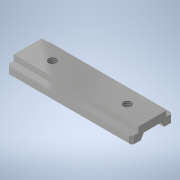
# Autodesk Inventor part: MR-20CS
Saved by Autodesk Inventor 2022 (Build 260153000, 153)
## iProperties
Created: 2022-02-08
Part Number: MR-20CS
Material: ポリエチレン、高密度
Document SubType Name: Modeling
Designer: satot
Density: 0.952 g/cm^3
Appearance: 滑らか - 標準の灰色
Mass: 2.70649 g
Surface Area: 24.218 cm^2
Volume: 2.84295 cm^3
Author: satot
Autodesk Inventor part; units mm, degrees
ref_plane "YZ Plane" through (0, 0, 0) normal (1, 0, 0) x (0, 1, 0)
ref_plane "XZ Plane" through (0, 0, 0) normal (0, 1, 0) x (-1, 0, 0)
ref_plane "XY Plane" through (0, 0, 0) normal (0, 0, 1) x (1, 0, 0)
sketch "スケッチ1" plane through (0, 0, 0) normal (0, 1, 0) x (-1, 0, 0)
  line L0 (-5.6, 0) -> (5.6, 0)
  line L1 (5.6, 0) -> (5.6, -2.2)
  line L2 (5.6, -2.2) -> (8.4, -2.2)
  line L3 (8.4, -2.2) -> (8.4, -5.2)
  line L4 (8.4, -5.2) -> (4.6551, -5.2)
  line L5 (4.6551, -5.2) -> (3.4551, -3.1215)
  line L6 (3.4551, -3.1215) -> (-3.4551, -3.1215)
  line L7 (-3.4551, -3.1215) -> (-4.6551, -5.2)
  line L8 (-4.6551, -5.2) -> (-8.4, -5.2)
  line L9 (-8.4, -5.2) -> (-8.4, -2.2)
  line L10 (-8.4, -2.2) -> (-5.6, -2.2)
  line L11 (-5.6, -2.2) -> (-5.6, 0)
  point P0 (0, 0)
  point P1 (0, 0)
  point P2 (0, -3.1215)
  dimension "d0" = 11.2
  dimension "d1" = 5.2
  dimension "d2" = 16.8
  dimension "d3" = 120
  dimension "d4" = 120
  dimension "d5" = 3
  constraints: 25 end point, 6 perpendicular, 4 point on line, 2 midpoint, 1 coincident, 1 collinear, 1 horizontal, 1 parallel, 1 vertical alignment
  measures "d0" distance of L0.start L0.end
  measures "d1" distance between parallel lines of L0 L4
  measures "d2" distance between parallel lines of L9 L3
  measures "d3" angle of L4 L5
  measures "d4" angle of L8 L7
  measures "d5" distance between parallel lines of L2 L4
extrude "押し出し1" add sketch "スケッチ1" along normal blind 50
chamfer "面取り1" [suppressed]
chamfer "面取り2" distance 1 angle 45 4 edges at (8.4, 0, -3.7) (-8.4, 0, -3.7) (8.4, 50, -3.7) (-8.4, 50, -3.7)
chamfer "面取り3" distance 0.3 angle 45 4 edges at (-8.4, 25, -2.2) (-8.4, 25, -5.2) (8.4, 25, -5.2) (8.4, 25, -2.2)
sketch "スケッチ2" plane through (-5.6, 0, 0) normal (0, 0, 1) x (1, 0, 0)
  line L0 (5.6, 10) -> (5.6, 40) construction
  line L1 (13.7, 49.3) -> (13.7, 0.7) construction
  line L2 (0, 0) -> (11.2, 0) construction
  point P0 (5.6, 0)
  point P1 (5.6, 25)
  point P2 (13.7, 25)
  point P3 (5.6, 0)
  dimension "d17" = 30
  constraints: 3 midpoint, 2 end point, 2 vertical alignment, 1 horizontal alignment, 1 vertical
  measures "d17" distance of L0.start L0.end
hole "穴1" at (0, 10, 0) at (0, 40, 0) direction (0, 0, -1) diameter 3.242 end through all thread size "M4x0.7" class "6H" standard "ANSI Metric M Profile"
